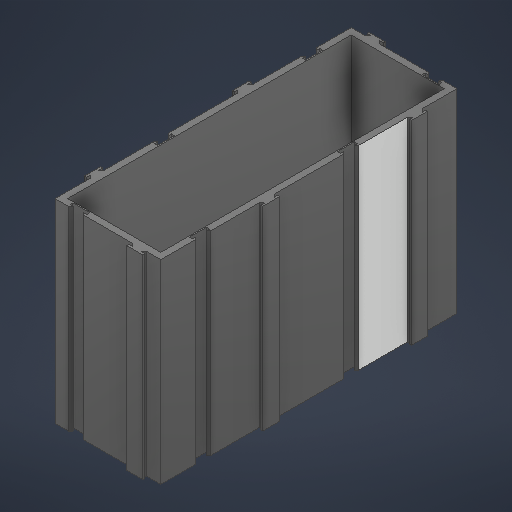
# Autodesk Inventor part: box2x1
Saved by Autodesk Inventor 2027 (Build 310192060, 192F)
## iProperties
Created: 2026-06-08
Part Number: box2x1
Material: Ogólny
Document SubType Name: Modeling
Designer: User
Density: 1 g/cm^3
Appearance: Domyślna
Author: User
Autodesk Inventor part; units mm, degrees
ref_plane "YZ Plane" through (0, 0, 0) normal (1, 0, 0) x (0, 1, 0)
ref_plane "XZ Plane" through (0, 0, 0) normal (0, 1, 0) x (-1, 0, 0)
ref_plane "XY Plane" through (0, 0, 0) normal (0, 0, 1) x (1, 0, 0)
sketch "Szkic1" plane through (0, 0, 0) normal (0, 1, 0) x (-1, 0, 0)
  line L0 (-25, -70) -> (25, -70)
  line L1 (25, -70) -> (25, 70)
  line L2 (25, 70) -> (-25, 70)
  line L3 (-25, 70) -> (-25, -70)
  line L4 (-25, -70) -> (25, 70) construction
  line L5 (25, -70) -> (-25, 70) construction
  line L6 (-22, -67) -> (22, -67)
  line L7 (22, -67) -> (22, 67)
  line L8 (22, 67) -> (-22, 67)
  line L9 (-22, 67) -> (-22, -67)
  line L10 (-22, -67) -> (22, 67) construction
  line L11 (22, -67) -> (-22, 67) construction
  line L12 (25, 70) -> (18.5607, 70)
  line L13 (25, 70) -> (31.4393, 70) construction
  line L14 (18.5607, 70) -> (17.5, 68.9393)
  line L15 (17.5, 68.9393) -> (19, 68.9393)
  line L16 (19, 68.9393) -> (19, 67.5393)
  line L17 (-25, 70) -> (-23, 70) construction
  line L18 (0, 67) -> (0, 70) construction
  line L19 (18.5607, 70) -> (32.6482, 70) construction
  line L20 (11.4393, 70) -> (29.6482, 70) construction
  line L21 (19, 67.5393) -> (15, 67.5393)
  line L22 (15, 67.5393) -> (15, 70) construction
  line L23 (11.4393, 70) -> (12.5, 68.9393)
  line L24 (12.5, 68.9393) -> (11, 68.9393)
  line L25 (11, 68.9393) -> (11, 67.5393)
  line L26 (11, 67.5393) -> (15, 67.5393)
  line L27 (-18.5607, 70) -> (-17.5, 68.9393) construction
  line L28 (-17.5, 68.9393) -> (-19, 68.9393) construction
  line L29 (-19, 67.5393) -> (-15, 67.5393) construction
  line L30 (-15, 67.5393) -> (-15, 70) construction
  line L31 (-11.4393, 70) -> (-12.5, 68.9393) construction
  line L32 (-11, 67.5393) -> (-15, 67.5393) construction
  line L33 (-11, 68.9393) -> (-11, 67.5393) construction
  line L34 (-12.5, 68.9393) -> (-11, 68.9393) construction
  line L35 (-19, 68.9393) -> (-19, 67.5393) construction
  line L36 (22, 0) -> (-22, 0) construction
  line L37 (25, 0) -> (22, 0) construction
  line L38 (18.5607, -70) -> (17.5, -68.9393) construction
  line L39 (17.5, -68.9393) -> (19, -68.9393) construction
  line L40 (19, -68.9393) -> (19, -67.5393) construction
  line L41 (19, -67.5393) -> (15, -67.5393) construction
  line L42 (15, -67.5393) -> (15, -70) construction
  line L43 (11.4393, -70) -> (12.5, -68.9393) construction
  line L44 (11, -67.5393) -> (15, -67.5393) construction
  line L45 (11, -68.9393) -> (11, -67.5393) construction
  line L46 (12.5, -68.9393) -> (11, -68.9393) construction
  line L47 (-11.4393, -70) -> (-12.5, -68.9393)
  line L48 (-12.5, -68.9393) -> (-11, -68.9393)
  line L49 (-15, -67.5393) -> (-15, -70) construction
  line L50 (-11, -67.5393) -> (-15, -67.5393)
  line L51 (-18.5607, -70) -> (-17.5, -68.9393)
  line L52 (-17.5, -68.9393) -> (-19, -68.9393)
  line L53 (-19, -67.5393) -> (-15, -67.5393)
  line L54 (-11, -68.9393) -> (-11, -67.5393)
  line L55 (-19, -68.9393) -> (-19, -67.5393)
  line L56 (25, 46.4393) -> (23.9393, 47.5) construction
  line L57 (23.9393, 47.5) -> (23.9393, 46) construction
  line L58 (23.9393, 46) -> (22.5393, 46) construction
  line L59 (22.5393, 46) -> (22.5393, 50) construction
  line L60 (22.5393, 50) -> (24.8, 50) construction
  line L61 (25, 53.5607) -> (23.9393, 52.5) construction
  line L62 (22.5393, 54) -> (22.5393, 50) construction
  line L63 (23.9393, 54) -> (22.5393, 54) construction
  line L64 (23.9393, 52.5) -> (23.9393, 54) construction
  line L65 (25, -46.4393) -> (23.9393, -47.5)
  line L66 (23.9393, -47.5) -> (23.9393, -46)
  line L67 (23.9393, -46) -> (22.5393, -46)
  line L68 (22.5393, -46) -> (22.5393, -50)
  line L69 (25, -53.5607) -> (23.9393, -52.5)
  line L70 (23.9393, -52.5) -> (23.9393, -54)
  line L71 (22.5393, -50) -> (24.8, -50) construction
  line L72 (22.5393, -54) -> (22.5393, -50)
  line L73 (23.9393, -54) -> (22.5393, -54)
  line L74 (-25, 46.4393) -> (-23.9393, 47.5)
  line L75 (-23.9393, 47.5) -> (-23.9393, 46)
  line L76 (-23.9393, 46) -> (-22.5393, 46)
  line L77 (-22.5393, 46) -> (-22.5393, 50)
  line L78 (-25, 53.5607) -> (-23.9393, 52.5)
  line L79 (-23.9393, 52.5) -> (-23.9393, 54)
  line L80 (-22.5393, 50) -> (-24.8, 50) construction
  line L81 (-22.5393, 54) -> (-22.5393, 50)
  line L82 (-23.9393, 54) -> (-22.5393, 54)
  line L83 (-25, -46.4393) -> (-23.9393, -47.5) construction
  line L84 (-23.9393, -47.5) -> (-23.9393, -46) construction
  line L85 (-23.9393, -46) -> (-22.5393, -46) construction
  line L86 (-22.5393, -46) -> (-22.5393, -50) construction
  line L87 (-22.5393, -50) -> (-24.8, -50) construction
  line L88 (-25, -53.5607) -> (-23.9393, -52.5) construction
  line L89 (-22.5393, -54) -> (-22.5393, -50) construction
  line L90 (-23.9393, -52.5) -> (-23.9393, -54) construction
  line L91 (-23.9393, -54) -> (-22.5393, -54) construction
  line L92 (-11.4393, 70) -> (-12.5, 71.0607)
  line L93 (-12.5, 71.0607) -> (-11, 71.0607)
  line L94 (-15, 72.4607) -> (-15, 70)
  line L95 (-11, 72.4607) -> (-15, 72.4607)
  line L96 (-18.5607, 70) -> (-17.5, 71.0607)
  line L97 (-17.5, 71.0607) -> (-19, 71.0607)
  line L98 (-19, 72.4607) -> (-15, 72.4607)
  line L99 (-11, 71.0607) -> (-11, 72.4607)
  line L100 (-19, 71.0607) -> (-19, 72.4607)
  line L101 (18.5607, -70) -> (17.5, -71.0607)
  line L102 (17.5, -71.0607) -> (19, -71.0607)
  line L103 (19, -71.0607) -> (19, -72.4607)
  line L104 (19, -72.4607) -> (15, -72.4607)
  line L105 (11, -72.4607) -> (15, -72.4607)
  line L106 (15, -72.4607) -> (15, -70) construction
  line L107 (11.4393, -70) -> (12.5, -71.0607)
  line L108 (11, -71.0607) -> (11, -72.4607)
  line L109 (12.5, -71.0607) -> (11, -71.0607)
  line L110 (25, 46.4393) -> (26.0607, 47.5)
  line L111 (26.0607, 47.5) -> (26.0607, 46)
  line L112 (26.0607, 46) -> (27.4607, 46)
  line L113 (27.4607, 46) -> (27.4607, 50)
  line L114 (25, 53.5607) -> (26.0607, 52.5)
  line L115 (26.0607, 52.5) -> (26.0607, 54)
  line L116 (27.4607, 50) -> (25.2, 50) construction
  line L117 (27.4607, 54) -> (27.4607, 50)
  line L118 (26.0607, 54) -> (27.4607, 54)
  line L119 (-26.0607, -54) -> (-27.4607, -54)
  line L120 (-26.0607, -52.5) -> (-26.0607, -54)
  line L121 (-25, -53.5607) -> (-26.0607, -52.5)
  line L122 (-27.4607, -46) -> (-27.4607, -50)
  line L123 (-27.4607, -50) -> (-25.2, -50) construction
  line L124 (-26.0607, -46) -> (-27.4607, -46)
  line L125 (-26.0607, -47.5) -> (-26.0607, -46)
  line L126 (-25, -46.4393) -> (-26.0607, -47.5)
  line L127 (-27.4607, -54) -> (-27.4607, -50)
  line L128 (25, -23.5807) -> (26.0607, -22.52)
  line L129 (26.0607, -22.52) -> (26.0607, -24.02)
  line L130 (26.0607, -24.02) -> (27.4607, -24.02)
  line L131 (27.4607, -24.02) -> (27.4607, -20.02)
  line L132 (26.0607, -16.02) -> (27.4607, -16.02)
  line L133 (26.0607, -17.52) -> (26.0607, -16.02)
  line L134 (25, -16.4593) -> (26.0607, -17.52)
  line L135 (27.4607, -20.02) -> (25.2, -20.02) construction
  line L136 (27.4607, -16.02) -> (27.4607, -20.02)
  line L137 (25, 23.5607) -> (23.9393, 22.5)
  line L138 (23.9393, 16) -> (22.5393, 16)
  line L139 (23.9393, 17.5) -> (23.9393, 16)
  line L140 (25, 16.4393) -> (23.9393, 17.5)
  line L141 (22.5393, 20) -> (24.8, 20) construction
  line L142 (23.9393, 22.5) -> (23.9393, 24)
  line L143 (22.5393, 16) -> (22.5393, 20)
  line L144 (22.5393, 24) -> (22.5393, 20)
  line L145 (23.9393, 24) -> (22.5393, 24)
  line L146 (-23.9393, -16) -> (-22.5393, -16)
  line L147 (-23.9393, -17.5) -> (-23.9393, -16)
  line L148 (-25, -16.4393) -> (-23.9393, -17.5)
  line L149 (-22.5393, -20) -> (-24.8, -20) construction
  line L150 (-25, -23.5607) -> (-23.9393, -22.5)
  line L151 (-23.9393, -24) -> (-22.5393, -24)
  line L152 (-23.9393, -22.5) -> (-23.9393, -24)
  line L153 (-26.0607, 24.02) -> (-27.4607, 24.02)
  line L154 (-27.4607, 24.02) -> (-27.4607, 20.02)
  line L155 (-27.4607, 20.02) -> (-25.2, 20.02) construction
  line L156 (-26.0607, 16.02) -> (-27.4607, 16.02)
  line L157 (-27.4607, 16.02) -> (-27.4607, 20.02)
  line L158 (-25, 23.5807) -> (-26.0607, 22.52)
  line L159 (-26.0607, 22.52) -> (-26.0607, 24.02)
  line L160 (-25, 16.4593) -> (-26.0607, 17.52)
  line L161 (-22.5393, -16) -> (-22.5393, -20)
  line L162 (-22.5393, -24) -> (-22.5393, -20)
  line L163 (-26.0607, 17.52) -> (-26.0607, 16.02)
  point P0 (0, 0)
  point P1 (-11.4393, 70)
  point P2 (-18.5607, 70)
  point P3 (-18.5607, -70)
  point P4 (-11.4393, -70)
  point P5 (11.4393, -70)
  point P6 (18.5607, -70)
  point P7 (0, 68.5)
  point P8 (15, 68.7697)
  point P9 (23.5, 0)
  point P10 (-15, 68.7697)
  point P11 (23.6697, 50)
  point P12 (23.6697, -50)
  point P13 (-23.6697, 50)
  point P14 (-23.6697, -50)
  point P15 (23.6697, -50)
  point P16 (-25, 53.5607)
  point P17 (-25, 46.4393)
  point P18 (-25, -46.4393)
  point P19 (-25, -53.5607)
  point P20 (25, -53.5607)
  point P21 (25, -46.4393)
  point P22 (-15, 71.2303)
  point P23 (26.3303, 50)
  point P24 (-26.3303, -50)
  point P25 (-25, -53.5607)
  point P26 (-25, -46.4393)
  point P27 (18.5607, -70)
  point P28 (11.4393, -70)
  point P29 (-18.5607, 70)
  point P30 (-11.4393, 70)
  point P31 (26.3303, -20.02)
  point P32 (23.6697, 20)
  point P33 (23.6697, 20)
  point P34 (-23.6697, -20)
  point P35 (-23.6697, -20)
  point P36 (-26.3303, 20.02)
  point P37 (25, -23.5807)
  point P38 (25, -16.4593)
  point P39 (-25, 16.4593)
  dimension "d0" = 50
  dimension "d1" = 140
  dimension "d2" = 44
  dimension "d3" = 134
  dimension "d6" = 1.5
  dimension "d7" = 135
  dimension "d8" = 1.5
  dimension "d9" = 1.4
  dimension "d15" = 2
  dimension "d23" = 4
  dimension "d29" = 45
  dimension "d34" = 1.5
  dimension "d35" = 1.5
  dimension "d36" = 1.4
  dimension "d37" = 4
  dimension "d38" = 45
  dimension "d76" = 1.1303
  dimension "d90" = 20
  dimension "d91" = 10
  dimension "d94" = 70.02
  dimension "d101" = 70
  dimension "d108" = 360
  constraints: 328 end point, 102 symmetric about line, 15 midpoint, 10 parallel, 7 point on line, 4 horizontal, 4 perpendicular, 4 vertical, 2 collinear, 122 other
  measures "d0" distance of L2.end L1.end
  measures "d1" distance of L1.end L0.end
  measures "d2" distance of L8.end L7.end
  measures "d3" distance of L7.end L6.end
  measures "d6" distance of L12.end L14.end
  measures "d7" angle of L14 L12
  measures "d8" distance of L14.end L15.end
  measures "d9" distance of L15.end L16.end
  measures "d15" distance of L2.end L17.end
  measures "d23" distance of L16.end L21.end
  measures "d29" angle of L24 L23
  measures "d34" distance of L56.start L56.end
  measures "d35" distance of L56.end L57.end
  measures "d36" distance of L57.end L58.end
  measures "d37" distance of L58.end L59.end
  measures "d38" angle of L64 L61
  measures "d76" distance of L68.end point (23.67, -50)
  measures "d90" distance from line of L2 point (23.67, 50)
  measures "d91" distance from line of L1 point (15, 68.77)
  measures "d94" distance of L111.start L128.end
  measures "d101" distance of L65.start L137.start
extrude "Wyciągnięcie proste1" add sketch "Szkic1" along normal blind 90 contours L3 L150 L152 L151 L162 L161 L146 L147 L148 L74 L75 L76 L77 L81 L82 L79 L78 L2 L23 L24 L25 L26 L21 L16 L15 L14 L1 L137 L142 L145 L144 L143 L138 L139 L140 L65 L66 L67 L68 L72 L73 L70 L69 L0 L47 L48 L54 L50 L53 L55 L52 L51 | L121 L120 L119 L127 L122 L124 L125 L126 L3 | L0 L101 L102 L103 L104 L105 L108 L109 L107 | L160 L163 L156 L157 L154 L153 L159 L158 L3 | L1 L134 L133 L132 L136 L131 L130 L129 L128 | L96 L97 L100 L98 L94 L2 | L94 L95 L99 L93 L92 L2 | L1 L114 L115 L118 L117 L113 L112 L111 L110
extrude "Wyciągnięcie proste2" add sketch "Szkic1" against normal blind 2 contours L3 L150 L152 L151 L162 L161 L146 L147 L148 L74 L75 L76 L77 L81 L82 L79 L78 L2 L23 L24 L25 L26 L21 L16 L15 L14 L1 L137 L142 L145 L144 L143 L138 L139 L140 L65 L66 L67 L68 L72 L73 L70 L69 L0 L47 L48 L54 L50 L53 L55 L52 L51 | L121 L120 L119 L127 L122 L124 L125 L126 L3 | L0 L101 L102 L103 L104 L105 L108 L109 L107 | L160 L163 L156 L157 L154 L153 L159 L158 L3 | L1 L134 L133 L132 L136 L131 L130 L129 L128 | L96 L97 L100 L98 L94 L2 | L94 L95 L99 L93 L92 L2 | L1 L114 L115 L118 L117 L113 L112 L111 L110 | L9 L8 L7 L6
offset faces "Rozmiar1" outward -0.2 faces at (-19, 59.3333, -71.5273) (-18.2071, 59.3333, -70.3536) (-16.3333, 59.3333, -72.4607) (-11, 59.3333, -71.994) (-12.1464, 59.3333, -70.7071) (-11.5, 59.3333, -71.0607) (-18, 59.3333, -71.0607) (-26.0607, 59.3333, 46.5) (-26.5273, 28.6667, 46) (-25.7071, 28.6667, 52.8536) (-26.994, 28.6667, 54) (-26.0607, 28.6667, 53.5) (-25.7071, 59.3333, 47.1464) (-27.4607, 28.6667, 48.6667) (13.6667, 28.6667, 72.4607) (19, 28.6667, 71.994) (17.8536, 28.6667, 70.7071) (18.5, 28.6667, 71.0607) (12, 28.6667, 71.0607) (11, 28.6667, 71.5273) (11.7929, 28.6667, 70.3536) (26.0607, 28.6667, -47) (26.994, 59.3333, -46) (27.4607, 59.3333, -51.3333) (26.5273, 59.3333, -54) (26.0607, 59.3333, -53) (-26.0607, 59.3333, -17.02) (-27.4607, 59.3333, -18.6867) (-26.0607, 59.3333, -23.52) (26.0607, 28.6667, 16.52) (26.0607, 28.6667, 23.02) (27.4607, 28.6667, 21.3533)
move faces "Przesuń1" translate (0.05, 0, 0) faces at (26.2607, 59.3333, -52.8) (26.2607, 28.6667, -47.2) (27.2607, 28.6667, -48.7333)
move faces "Przesuń2" translate (-0.05, 0, 0) faces at (-26.2607, 59.3333, 52.6114) (-26.2607, 59.3333, 46.7943) (-27.2607, 59.3333, 51.2667)
move faces "Przesuń3" translate (0, 0, -0.05) faces at (-11.7943, 59.3333, -71.2607) (-17.6114, 59.3333, -71.2607) (-16.2667, 59.3333, -72.2607)
move faces "Przesuń4" translate (0, 0, 0.05) faces at (16.2667, 59.3333, 72.2607) (17.6114, 59.3333, 71.2607) (11.7943, 59.3333, 71.2607)
equation "\"Offcenter\" = 15"
